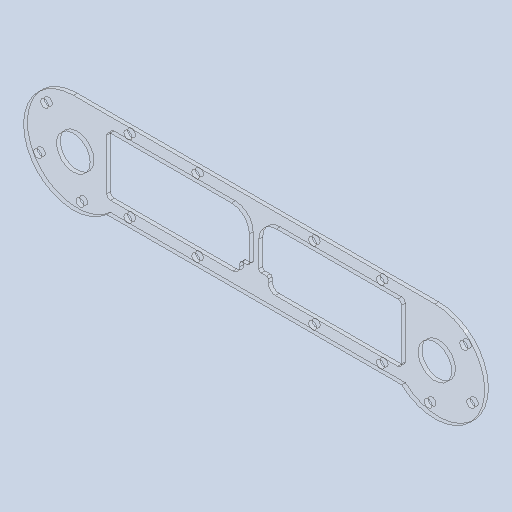
# Autodesk Inventor part: Mech Panel v7 skin interior
Saved by Autodesk Inventor 2022 (Build 260153000, 153)
## iProperties
Created: 2022-09-25
Part Number: Mech Panel v7 skin interior
Material: Polycarbonate, Clear
Document SubType Name: Modeling
Designer: matt
Density: 1.2 g/cm^3
Appearance: Polycarbonate - Clear
Mass: 74.4411 g
Surface Area: 457.903 cm^2
Volume: 62.0342 cm^3
Author: matt
Autodesk Inventor part; units mm, degrees
ref_plane "YZ Plane" through (0, 0, 0) normal (1, 0, 0) x (0, 1, 0)
ref_plane "XZ Plane" through (0, 0, 0) normal (0, 1, 0) x (-1, 0, 0)
ref_plane "XY Plane" through (0, 0, 0) normal (0, 0, 1) x (1, 0, 0)
sketch "Sketch3" plane through (0, 0, 0) normal (0, 0, 1) x (1, 0, 0)
  line L0 (-148.6937, 15) -> (-148.6937, 3.447)
  line L1 (-28.1723, 30) -> (-145.5187, 30)
  line L2 (-137.6119, -19.15) -> (-31.3473, -19.15)
  line L3 (-137.6488, -19.15) -> (-137.6119, -19.15)
  line L4 (-139.747, -0.553) -> (-139.747, -13.15)
  arc A0 (-139.747, -0.553) -> (-142.2077, 1.447) centre (-141.7463, -0.4991) ccw
  line L5 (-146.6937, 1.447) -> (-142.2077, 1.447)
  arc A1 (-148.6937, 3.447) -> (-146.6937, 1.447) centre (-146.6937, 3.447) ccw
  circle A2 centre (24.2686, 23.8125) radius 3.35
  circle A3 centre (30.1464, -15.7223) radius 3.35
  circle A4 centre (-5.6371, -33.5294) radius 3.35
  circle A5 centre (-46.0375, 36) radius 3.35
  circle A6 centre (-46.0375, -25.15) radius 3.35
  line L6 (-152.6937, -31.15) -> (-152.6937, 42) construction
  line L7 (-28.1723, -31.15) -> (-152.6937, -31.15)
  arc A7 (-28.1723, -31.15) -> (0, 42) centre (0, 0) ccw
  line L8 (-152.6937, 42) -> (0, 42)
  circle A8 centre (0, 0) radius 14.224
  line L9 (-31.3473, 30) -> (-133.6937, 30)
  line L10 (-148.6937, 26.825) -> (-148.6937, -19.15)
  line L11 (-133.747, -19.15) -> (-28.1723, -19.15)
  line L12 (-28.1723, -15.975) -> (-28.1723, 26.825)
  arc A9 (-28.1723, 26.825) -> (-31.3473, 30) centre (-31.3473, 26.825) ccw
  arc A10 (-31.3473, -19.15) -> (-28.1723, -15.975) centre (-31.3473, -15.975) ccw
  line L13 (-165.6403, -0.553) -> (-165.6403, -13.15)
  arc A11 (-163.1796, 1.447) -> (-165.6403, -0.553) centre (-163.641, -0.4991) ccw
  line L14 (-158.6937, 1.447) -> (-163.1796, 1.447)
  arc A12 (-158.6937, 1.447) -> (-156.6937, 3.447) centre (-158.6937, 3.447) ccw
  line L15 (-156.6937, 26.825) -> (-156.6937, 3.447)
  line L16 (-277.2151, -31.15) -> (-152.6937, -31.15)
  line L17 (-152.6937, 42) -> (-305.3873, 42)
  line L18 (-277.2151, 30) -> (-159.8687, 30)
  line L19 (-167.7755, -19.15) -> (-274.0401, -19.15)
  circle A13 centre (-259.3498, 36) radius 3.35
  circle A14 centre (-259.3498, -25.15) radius 3.35
  circle A15 centre (-299.7503, -33.5294) radius 3.35
  arc A16 (-305.3873, 42) -> (-277.2151, -31.15) centre (-305.3873, 0) ccw
  circle A17 centre (-329.6559, 23.8125) radius 3.35
  circle A18 centre (-335.5338, -15.7223) radius 3.35
  circle A19 centre (-305.3873, 0) radius 14.224
  line L20 (-274.0401, 30) -> (-171.6937, 30)
  line L21 (-156.6937, 15) -> (-156.6937, -19.15)
  line L22 (-171.6403, -19.15) -> (-277.2151, -19.15)
  line L23 (-277.2151, -15.975) -> (-277.2151, 26.825)
  arc A20 (-274.0401, 30) -> (-277.2151, 26.825) centre (-274.0401, 26.825) ccw
  arc A21 (-277.2151, -15.975) -> (-274.0401, -19.15) centre (-274.0401, -15.975) ccw
  arc A22 (-156.6937, 26.825) -> (-159.8687, 30) centre (-159.8687, 26.825) ccw
  circle A23 centre (-103.364, 36) radius 3.35
  circle A24 centre (-202.0233, 36) radius 3.35 projected
  circle A25 centre (-202.0233, -25.15) radius 3.35 projected
  circle A26 centre (-103.364, -25.15) radius 3.35 projected
  line L24 (-148.6937, 19.85) -> (-19.7478, 19.85) projected
  line L25 (-148.6937, 28) -> (-148.6937, 19.85) projected
  arc A27 (-146.6937, 30) -> (-148.6937, 28) centre (-146.6937, 28) ccw projected
  line L26 (0, 30) -> (-146.6937, 30) projected
  line L27 (0, 28) -> (0, 30) projected
  arc A28 (0, 28) -> (-19.7478, 19.85) centre (0, 0) ccw projected
  line L28 (-156.6937, 19.85) -> (-285.6395, 19.85) projected
  arc A29 (-285.6395, 19.85) -> (-305.3873, 28) centre (-305.3873, 0) ccw projected
  line L29 (-305.3873, 28) -> (-305.3873, 30) projected
  line L30 (-305.3873, 30) -> (-158.6937, 30) projected
  arc A30 (-156.6937, 28) -> (-158.6937, 30) centre (-158.6937, 28) ccw projected
  line L31 (-156.6937, 28) -> (-156.6937, 19.85) projected
  arc A31 (-133.6937, 30) -> (-148.6937, 15) centre (-133.6937, 15) ccw
  arc A32 (-156.6937, 15) -> (-171.6937, 30) centre (-171.6937, 15) ccw
  line L32 (-148.6937, 1.447) -> (-141.747, 1.447) projected
  line L33 (-139.747, -0.553) -> (-139.747, -13.15) projected
  arc A33 (-139.747, -13.15) -> (-133.747, -19.15) centre (-133.747, -13.15) ccw
  arc A34 (-171.6403, -19.15) -> (-165.6403, -13.15) centre (-171.6403, -13.15) ccw
  arc A35 (-140.7256, -13.15) -> (-134.7256, -19.15) centre (-134.7256, -13.15) ccw projected
  line L34 (-140.7256, -10.1131) -> (-140.7256, -13.15) projected
  arc A36 (-140.7256, -10.1131) -> (-142.2077, -8.6311) centre (-142.2077, -10.1131) ccw projected
  line L35 (-152.6937, -8.6311) -> (-142.2077, -8.6311) projected
  arc A37 (-148.6937, -6.6311) -> (-146.6937, -8.6311) centre (-146.6937, -6.6311) ccw projected
  arc A38 (-158.6937, -8.6311) -> (-156.6937, -6.6311) centre (-158.6937, -6.6311) ccw projected
  line L36 (-152.6937, -8.6311) -> (-163.1796, -8.6311) projected
  arc A39 (-163.1796, -8.6311) -> (-164.6617, -10.1131) centre (-163.1796, -10.1131) ccw projected
  line L37 (-164.6617, -10.1131) -> (-164.6617, -13.15) projected
  arc A40 (-170.6617, -19.15) -> (-164.6617, -13.15) centre (-170.6617, -13.15) ccw projected
  point P0 (-139.747, -14.6539)
  point P1 (-148.6937, 13.3123)
  point P2 (-31.3473, 30)
  point P3 (-31.3473, -19.15)
  point P4 (-137.6488, -19.0723)
  point P5 (-148.6937, 3.447)
  point P6 (-165.6403, -14.6539)
  point P7 (-274.0401, -19.15)
  point P8 (-156.6937, 3.447)
  point P9 (-137.6488, -19.15)
  dimension "d8" = 28.448
  dimension "d9" = 3.175
  dimension "d16" = 6.7
  dimension "d17" = 6.7
  dimension "d18" = 15
  dimension "d19" = 6
  dimension "d20" = 6
  constraints: 46 end point, 30 point on circle, 30 symmetric about line, 28 centre point, 15 point on line, 12 tangent, 4 collinear, 2 equal radius, 2 parallel, 1 horizontal, 1 perpendicular, 16 other
  measures "d8" diameter of A8
  measures "d9" radius of A9
  measures "d16" diameter of A23
  measures "d17" diameter of A24
  measures "d18" radius of A31
  measures "d19" radius of A33
  measures "d20" radius of A34
extrude "Extrusion3" add sketch "Sketch3" along normal blind 3.175 contours L36 A38 L21 | L10 L24 A31 | L10 L25 A27 L26 L1 A31 L24 | L12 A9 L1 L26 L27 A28 L24 | A37 L35 L10 | A32 L28 L15 | L28 A32 L18 A22 L15 | A22 L30 A30 L31 | L28 A29 L29 L30 L18 A20 L23 | L7 L16 A16 L17 L8 A7
body "Solid3"
